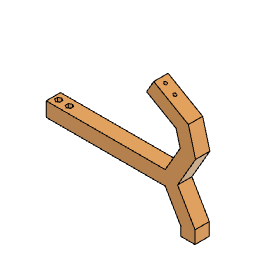
leg (Autodesk Fusion 360 design; units mm, degrees)
Autodesk Fusion 360 part; units mm, degrees
sketch "Sketch1" plane through (0, 0, 0) normal (0, 1, 0) x (1, 0, 0)
  line L0 (0, 0) -> (44.8288, 25.8819)
  line L1 (0, 0) -> (68.1027, 0) construction
  line L2 (44.8288, 25.8819) -> (52.6768, 55.1712)
  line L3 (52.6768, 55.1712) -> (26.7949, 100)
  line L4 (26.7949, 100) -> (52.6768, 144.8288)
  line L5 (26.7949, 100) -> (-145.5051, 100)
  line L6 (0, 0) -> (26.7949, 100) construction
  circle A0 centre (13.3975, 50) radius 36.6025 construction
  line L7 (52.6768, 144.8288) -> (52.6768, 160)
  dimension "d1" = 30
  dimension "d2" = 120
  dimension "d3" = 120
  dimension "d4" = 135
  dimension "d5" = 100
  dimension "d29" = 60
  dimension "d30" = 172.3
  constraint coincident L0.start L1.start
  constraint horizontal L1
  constraint horizontal L5
  constraint equal L0 L3
  constraint midpoint L6 A0.centre
  constraint tangent L0 A0
  constraint tangent L2 A0
  constraint vertical L2.end L4.end
  constraint vertical L7
  measures "d1" angle of L0 L1
  measures "d2" angle of L3 L4
  measures "d3" angle of L4 L5
  measures "d4" angle of L0 L2
  measures "d5" distance of L0.start L5
  measures "d29" distance of L5 L7.end
  measures "d30" distance of L3.end L5.end
pipe "Pipe1" add square section size 20 path "Sketch1" along L0 L2 L3 L4 L7
pipe "Pipe2" add square section size 20 path "Sketch1" along L5
sketch "Sketch2" plane through (5, 0, 8.6603) normal (0.5, 0, 0.866025) x (0, 1, 0)
  line L0 (10, 0) -> (-10, 0)
  line L1 (-10, 0) -> (-10, -55.9059)
  line L2 (-10, -55.9059) -> (10, -55.9059)
  line L3 (10, -55.9059) -> (10, 0)
  line L4 (0, 0) -> (0, -55.9059) construction
  circle A0 centre (0, -7.5) radius 2
  circle A1 centre (0, -22.5) radius 2
  line L5 (2.1362, -3.8) -> (-2.1362, -3.8)
  line L6 (-2.1362, -3.8) -> (-4.2724, -7.5)
  line L7 (-4.2724, -7.5) -> (-2.1362, -11.2)
  line L8 (-2.1362, -11.2) -> (2.1362, -11.2)
  line L9 (2.1362, -11.2) -> (4.2724, -7.5)
  line L10 (4.2724, -7.5) -> (2.1362, -3.8)
  line L11 (2.1362, -18.8) -> (-2.1362, -18.8)
  line L12 (-2.1362, -18.8) -> (-4.2724, -22.5)
  line L13 (-4.2724, -22.5) -> (-2.1362, -26.2)
  line L14 (-2.1362, -26.2) -> (2.1362, -26.2)
  line L15 (2.1362, -26.2) -> (4.2724, -22.5)
  line L16 (4.2724, -22.5) -> (2.1362, -18.8)
  point P0 (0, -7.5)
  point P1 (0, -22.5)
  dimension "d14" = 4
  dimension "d15" = 7.5
  dimension "d16" = 15
  dimension "d19" = 7.4
  constraint coincident L4.start origin
  constraint midpoint L2 L4.end
  constraint coincident L4 P0
  constraint coincident L4 P1
  constraint equal A0 A1
  constraint coincident P0 A0.centre
  constraint coincident P1 A1.centre
  constraint horizontal L5.start L5.end
  constraint horizontal L11
  constraint vertical L9.end L15.end
  measures "d14" diameter of A0
  measures "d15" distance of L4.start A0.centre
  measures "d16" distance of P0 P1
  measures "d19" distance of L5.start L8.end
extrude "Extrude1" cut sketch "Sketch2" against normal blind 35 contours A0 | A1
extrude "Extrude2" cut sketch "Sketch2" along normal blind 5 from surface at -20 contours L5 L6 L7 L8 L9 L10 | L11 L12 L13 L14 L15 L16
sketch "Sketch3" plane through (0, -10, 0) normal (0, -1, 0) x (1, 0, 0)
  line L0 (21.0214, -90) -> (-145.5051, -90)
  line L1 (-145.5051, -90) -> (-145.5051, -110)
  line L2 (-145.5051, -110) -> (21.0214, -110)
  line L3 (21.0214, -110) -> (42.6768, -147.5083)
  line L4 (42.6768, -160) -> (62.6768, -160)
  line L5 (62.6768, -142.1493) -> (38.3419, -100)
  line L6 (38.3419, -100) -> (63.4081, -56.584)
  line L7 (63.4081, -56.584) -> (53.416, -19.2927)
  line L8 (53.416, -19.2927) -> (5, 8.6603)
  line L9 (5, 8.6603) -> (-5, -8.6603)
  line L10 (-5, -8.6603) -> (36.2416, -32.4711)
  line L11 (36.2416, -32.4711) -> (41.9455, -53.7584)
  line L12 (41.9455, -53.7584) -> (21.0214, -90)
  line L13 (49.8889, -160) -> (82.45, -160)
  line L14 (82.45, -160) -> (110.5593, -200.6722)
  line L15 (110.5593, -200.6722) -> (43.8339, -200.6722)
  line L16 (43.8339, -200.6722) -> (49.8889, -160)
  line L17 (67.2094, -160) -> (67.2094, -150)
  line L18 (42.6768, -147.5083) -> (42.6768, -160)
  line L19 (62.6768, -160) -> (62.6768, -142.1493)
  dimension "d24" = 50
  dimension "d28" = 10
  constraint coincident L3 L13.start
  constraint horizontal L13
  constraint parallel L13 L15
  constraint coincident L13 L17.start
  constraint coincident L5 L17.end
  constraint perpendicular L13 L17
  measures "d24" vertical distance of L2.end L13.start
  measures "d28" distance of L17.start L17.end
sketch "Sketch4" plane through (0, 0, -90) normal (0, 0, 1) x (-1, 0, 0)
  line L0 (-21.0214, 10) -> (-21.0214, -10)
  line L1 (-21.0214, -10) -> (145.5051, -10)
  line L2 (145.5051, -10) -> (145.5051, 10)
  line L3 (145.5051, 10) -> (-21.0214, 10)
  line L4 (145.5051, 0) -> (43.2223, 0) construction
  circle A0 centre (138.0051, 0) radius 2
  circle A1 centre (123.0051, 0) radius 2
  line L5 (141.7051, -2.1362) -> (141.7051, 2.1362)
  line L6 (141.7051, 2.1362) -> (138.0051, 4.2724)
  line L7 (138.0051, 4.2724) -> (134.3051, 2.1362)
  line L8 (134.3051, 2.1362) -> (134.3051, -2.1362)
  line L9 (134.3051, -2.1362) -> (138.0051, -4.2724)
  line L10 (138.0051, -4.2724) -> (141.7051, -2.1362)
  line L11 (126.7051, -2.1362) -> (126.7051, 2.1362)
  line L12 (126.7051, 2.1362) -> (123.0051, 4.2724)
  line L13 (123.0051, 4.2724) -> (119.3051, 2.1362)
  line L14 (119.3051, 2.1362) -> (119.3051, -2.1362)
  line L15 (119.3051, -2.1362) -> (123.0051, -4.2724)
  line L16 (123.0051, -4.2724) -> (126.7051, -2.1362)
  point P0 (138.0051, 0)
  point P1 (123.0051, 0)
  dimension "d31" = 4
  dimension "d32" = 7.5
  dimension "d33" = 15
  dimension "d34" = 7.4
  constraint midpoint L2 L4.start
  constraint perpendicular L2 L4
  constraint coincident L4 P0
  constraint coincident L4 P1
  constraint equal A0 A1
  constraint coincident P0 A0.centre
  constraint coincident P1 A1.centre
  constraint vertical L5
  constraint vertical L11
  constraint horizontal L9.end L15.end
  measures "d31" diameter of A0
  measures "d32" distance of L4.start P0
  measures "d33" distance of P0 P1
  measures "d34" distance of L5 L8
extrude "Extrude4" cut sketch "Sketch4" against normal blind 50 contours A0 | A1
extrude "Extrude5" cut sketch "Sketch4" against normal blind 5 contours L5 L6 L7 L8 L9 L10 | L11 L12 L13 L14 L15 L16
equation "d19 = 7 mm + 2 * gap"
equation "gap = 0.2 mm"
equation "d34 = 7 mm + 2 * gap"
